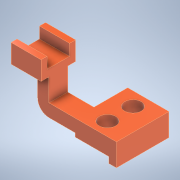
# Autodesk Inventor part: 051665019_14
Saved by Autodesk Inventor 2021 (Build 250183000, 183)
## iProperties
Created: 2020-05-26
Part Number: 051665019_14
Material: Generic
Document SubType Name: Modeling
Designer: figen
Density: 1 g/cm^3
Appearance: Smooth - Light Orange
Author: figen
Autodesk Inventor part; units mm, degrees
ref_plane "YZ Plane" through (0, 0, 0) normal (1, 0, 0) x (0, 1, 0)
ref_plane "XZ Plane" through (0, 0, 0) normal (0, 1, 0) x (-1, 0, 0)
ref_plane "XY Plane" through (0, 0, 0) normal (0, 0, 1) x (1, 0, 0)
sketch "Sketch1" plane through (0, 0, 0) normal (0, 0, 1) x (1, 0, 0)
  line L0 (0, 0) -> (-100, 0)
  line L1 (-100, 0) -> (-100, 80)
  line L2 (-100, 80) -> (-550, 80)
  line L3 (-550, 80) -> (-550, 130)
  line L4 (-550, 130) -> (-1050, 130)
  line L5 (-1050, 130) -> (-1050, 600)
  line L6 (-1050, 600) -> (-900, 600)
  line L7 (-900, 600) -> (-900, 300)
  line L8 (-900, 300) -> (0, 300)
  line L9 (0, 300) -> (0, 0)
  line L10 (-550, 130) -> (-550, 300)
  dimension "d0" = 100
  dimension "d1" = 80
  dimension "d2" = 450
  dimension "d3" = 50
  dimension "d4" = 500
  dimension "d5" = 470
  dimension "d6" = 150
  dimension "d7" = 300
  constraints: 22 end point, 9 perpendicular, 1 horizontal, 1 point on line, 1 vertical
  measures "d0" distance of L0.start L0.end
  measures "d1" distance of L0.end L1.end
  measures "d2" distance of L1.end L2.end
  measures "d3" distance of L2.end L3.end
  measures "d4" distance of L3.end L4.end
  measures "d5" distance of L4.end L5.end
  measures "d6" distance of L5.end L6.end
  measures "d7" distance of L6.end L7.end
extrude "Extrusion1" add sketch "Sketch1" against normal blind 700 contours L0 L1 L2 L3 L10 L8 L9
sketch "Sketch2" plane through (0, 0, 0) normal (0, 0, 1) x (1, 0, 0)
  line L0 (-100, 80) -> (-550, 80) construction
  line L1 (-550, 80) -> (-550, 130)
  line L2 (-550, 80) -> (-550, 300) construction
  line L3 (-550, 130) -> (-1050, 130)
  line L4 (-1050, 130) -> (-1050, 600)
  line L5 (-1050, 600) -> (-900, 600)
  line L6 (-900, 600) -> (-900, 300)
  line L7 (-900, 300) -> (-550, 300)
  line L8 (-550, 300) -> (-550, 80) construction
  line L9 (-550, 130) -> (-550, 300)
  point P0 (0, 0)
  dimension "d10" = 50
  dimension "d11" = 500
  dimension "d12" = 470
  dimension "d13" = 150
  dimension "d14" = 300
  constraints: 14 end point, 4 perpendicular, 1 point on line, 1 vertical
  measures "d10" distance of L0.end L1.end
  measures "d11" distance of L1.end L3.end
  measures "d12" distance of L3.end L4.end
  measures "d13" distance of L4.end L5.end
  measures "d14" distance of L5.end L6.end
extrude "Extrusion2" add sketch "Sketch2" against normal blind 250
sketch "Sketch3" plane through (-900, 300, 0) normal (1, 0, 0) x (0, 0, -1)
  line L0 (0, 300) -> (250, 300) construction
  line L1 (0, 300) -> (-105, 300)
  line L2 (-105, 300) -> (-105, 550)
  line L3 (-105, 550) -> (-25, 550)
  line L4 (-25, 550) -> (-25, 400)
  line L5 (-25, 400) -> (275, 400)
  line L6 (275, 400) -> (275, 550)
  line L7 (275, 550) -> (355, 550)
  line L8 (355, 550) -> (355, 300)
  line L9 (355, 300) -> (0, 300)
  point P0 (0, -300)
  dimension "d17" = 105
  dimension "d18" = 250
  dimension "d19" = 80
  dimension "d20" = 150
  dimension "d21" = 300
  dimension "d22" = 80
  constraints: 18 end point, 6 perpendicular, 3 point on line, 1 collinear, 1 horizontal
  measures "d17" distance of L0.start L1.end
  measures "d18" distance of L1.end L2.end
  measures "d19" distance of L2.end L3.end
  measures "d20" distance of L3.end L4.end
  measures "d21" distance of L4.end L5.end
  measures "d22" distance of L6.end L7.end
extrude "Extrusion3" add sketch "Sketch3" against normal blind 400
fillet "Fillet1" radius 150 1 edges at (-1050, 130, -125)
sketch "Sketch4" plane through (-550, 300, -700) normal (0, 1, 0) x (1, 0, 0)
  line L0 (450, -700) -> (550, -700) construction
  line L1 (550, -700) -> (550, -520)
  line L2 (550, -520) -> (250, -520)
  line L3 (250, -520) -> (250, -180)
  circle A0 centre (250, -520) radius 110
  circle A1 centre (250, -180) radius 110
  dimension "d26" = 180
  dimension "d27" = 300
  dimension "d28" = 340
  dimension "d29" = 220
  dimension "d30" = 220
  constraints: 6 end point, 2 centre point, 2 coincident, 2 perpendicular, 1 vertical
  measures "d26" distance of L0.end L1.end
  measures "d27" distance of L1.end L2.end
  measures "d28" distance of L2.end L3.end
  measures "d29" diameter of A0
  measures "d30" diameter of A1
extrude "Extrusion4" cut sketch "Sketch4" against normal blind 449.2125
body "Solid1"
